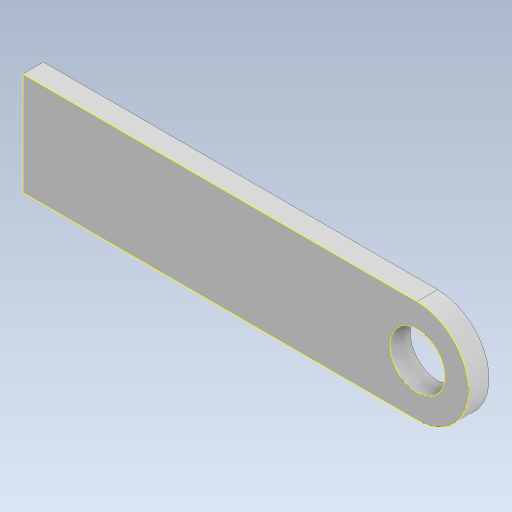
# Autodesk Inventor part: 零件6
Saved by Autodesk Inventor 2023 (Build 270158000, 158)
## iProperties
Created: 2023-05-12
Part Number: 零件6
Material: 一般
Document SubType Name: Modeling
Designer: Johnny Jou
Density: 1 g/cm^3
Appearance: 預設
Author: Johnny Jou
Autodesk Inventor part; units mm, degrees
ref_plane "YZ Plane" through (0, 0, 0) normal (1, 0, 0) x (0, 1, 0)
ref_plane "XZ Plane" through (0, 0, 0) normal (0, 1, 0) x (-1, 0, 0)
ref_plane "XY Plane" through (0, 0, 0) normal (0, 0, 1) x (1, 0, 0)
sketch "草圖1" plane through (0, 0, 0) normal (0, 0, 1) x (1, 0, 0)
  line L0 (0, 0) -> (50, 0)
  line L1 (50, 0) -> (50, 15)
  line L2 (50, 15) -> (0, 15)
  line L3 (0, 15) -> (0, 0)
  circle A0 centre (57.5, 7.5) radius 7.5
  line L4 (50, 15) -> (57.5, 15)
  line L5 (50, 0) -> (57.5, 0)
  circle A1 centre (57.5, 7.5) radius 4
  dimension "d0" = 50
  dimension "d1" = 15
  dimension "d2" = 15
  dimension "d3" = 8
  constraints: 12 end point, 4 tangent, 2 centre point, 2 parallel, 2 point on circle, 1 coincident, 1 horizontal, 1 perpendicular
  measures "d0" distance of L1.end L2.end
  measures "d1" distance of L0.end L1.end
  measures "d2" diameter of A0
  measures "d3" diameter of A1
extrude "擠出1" add sketch "草圖1" along normal blind 3
sketch "草圖2" plane through (0, 0, 3) normal (0, 0, 1) x (1, 0, 0)
  line L0 (0, 0) -> (57.5, 0) projected
  arc A0 (57.5, 0) -> (57.5, 15) centre (57.5, 7.5) ccw projected
  line L1 (57.5, 15) -> (0, 15) projected
  line L2 (0, 15) -> (0, 0) projected
  circle A1 centre (57.5, 7.5) radius 4 projected
